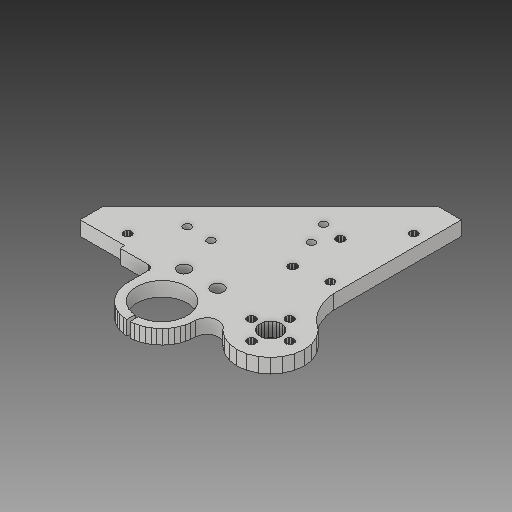
# Autodesk Inventor part: Left Bed Holder Lower
Saved by Autodesk Inventor 2018 (Build 220112000, 112)
## iProperties
Created: 2016-07-12
Part Number: Left Bed Holder Lower
Material: Generic
Document SubType Name: Modeling
Designer: joshmamo
Density: 1 g/cm^3
Appearance: Default
Author: joshmamo
Autodesk Inventor part; units mm, degrees
ref_plane "YZ Plane" through (0, 0, 0) normal (1, 0, 0) x (0, 1, 0)
ref_plane "XZ Plane" through (0, 0, 0) normal (0, 1, 0) x (-1, 0, 0)
ref_plane "XY Plane" through (0, 0, 0) normal (0, 0, 1) x (1, 0, 0)
sketch "Sketch2" plane through (0, 0, 0) normal (0, 1, 0) x (-1, 0, 0)
  line L0 (42.8996, 849.7412) -> (43.4826, 850.761)
  line L1 (43.4826, 850.761) -> (44.3097, 851.5953)
  line L2 (44.3097, 851.5953) -> (45.3245, 852.187)
  line L3 (45.3245, 852.187) -> (46.4579, 852.4959)
  line L4 (46.4579, 852.4959) -> (47.6326, 852.501)
  line L5 (47.6326, 852.501) -> (48.7686, 852.2018)
  line L6 (48.7686, 852.2018) -> (49.7885, 851.6188)
  line L7 (49.7885, 851.6188) -> (50.6227, 850.7917)
  line L8 (50.6227, 850.7917) -> (51.2145, 849.7769)
  line L9 (51.2145, 849.7769) -> (51.5234, 848.6435)
  line L10 (51.5234, 848.6435) -> (51.5284, 847.4688)
  line L11 (51.5284, 847.4688) -> (51.2293, 846.3328)
  line L12 (51.2293, 846.3328) -> (50.6463, 845.3129)
  line L13 (50.6463, 845.3129) -> (49.8192, 844.4787)
  line L14 (49.8192, 844.4787) -> (48.8044, 843.887)
  line L15 (48.8044, 843.887) -> (47.671, 843.578)
  line L16 (47.671, 843.578) -> (46.4963, 843.573)
  line L17 (46.4963, 843.573) -> (45.3603, 843.8722)
  line L18 (45.3603, 843.8722) -> (44.3404, 844.4551)
  line L19 (44.3404, 844.4551) -> (43.5062, 845.2822)
  line L20 (43.5062, 845.2822) -> (42.9144, 846.297)
  line L21 (42.9144, 846.297) -> (42.6055, 847.4304)
  line L22 (42.6055, 847.4304) -> (42.6005, 848.6052)
  line L23 (42.6005, 848.6052) -> (42.8996, 849.7412)
  line L24 (39.0644, 849.737) -> (39.5044, 849.6791)
  line L25 (39.5044, 849.6791) -> (39.9144, 849.5092)
  line L26 (39.9144, 849.5092) -> (40.2665, 849.2391)
  line L27 (40.2665, 849.2391) -> (40.5367, 848.887)
  line L28 (40.5367, 848.887) -> (40.7065, 848.477)
  line L29 (40.7065, 848.477) -> (40.7644, 848.037)
  line L30 (40.7644, 848.037) -> (40.7065, 847.597)
  line L31 (40.7065, 847.597) -> (40.5367, 847.187)
  line L32 (40.5367, 847.187) -> (40.2665, 846.8349)
  line L33 (40.2665, 846.8349) -> (39.9144, 846.5647)
  line L34 (39.9144, 846.5647) -> (39.5044, 846.3949)
  line L35 (39.5044, 846.3949) -> (39.0644, 846.337)
  line L36 (39.0644, 846.337) -> (38.6245, 846.3949)
  line L37 (38.6245, 846.3949) -> (38.2144, 846.5647)
  line L38 (38.2144, 846.5647) -> (37.8624, 846.8349)
  line L39 (37.8624, 846.8349) -> (37.5922, 847.187)
  line L40 (37.5922, 847.187) -> (37.4224, 847.597)
  line L41 (37.4224, 847.597) -> (37.3644, 848.037)
  line L42 (37.3644, 848.037) -> (37.4224, 848.477)
  line L43 (37.4224, 848.477) -> (37.5922, 848.887)
  line L44 (37.5922, 848.887) -> (37.8624, 849.2391)
  line L45 (37.8624, 849.2391) -> (38.2144, 849.5092)
  line L46 (38.2144, 849.5092) -> (38.6245, 849.6791)
  line L47 (38.6245, 849.6791) -> (39.0644, 849.737)
  line L48 (55.0644, 846.337) -> (54.6245, 846.3949)
  line L49 (54.6245, 846.3949) -> (54.2144, 846.5647)
  line L50 (54.2144, 846.5647) -> (53.8624, 846.8349)
  line L51 (53.8624, 846.8349) -> (53.5922, 847.187)
  line L52 (53.5922, 847.187) -> (53.4224, 847.597)
  line L53 (53.4224, 847.597) -> (53.3644, 848.037)
  line L54 (53.3644, 848.037) -> (53.4224, 848.477)
  line L55 (53.4224, 848.477) -> (53.5922, 848.887)
  line L56 (53.5922, 848.887) -> (53.8624, 849.2391)
  line L57 (53.8624, 849.2391) -> (54.2144, 849.5092)
  line L58 (54.2144, 849.5092) -> (54.6245, 849.6791)
  line L59 (54.6245, 849.6791) -> (55.0644, 849.737)
  line L60 (55.0644, 849.737) -> (55.5044, 849.6791)
  line L61 (55.5044, 849.6791) -> (55.9144, 849.5092)
  line L62 (55.9144, 849.5092) -> (56.2665, 849.2391)
  line L63 (56.2665, 849.2391) -> (56.5367, 848.887)
  line L64 (56.5367, 848.887) -> (56.7065, 848.477)
  line L65 (56.7065, 848.477) -> (56.7644, 848.037)
  line L66 (56.7644, 848.037) -> (56.7065, 847.597)
  line L67 (56.7065, 847.597) -> (56.5367, 847.187)
  line L68 (56.5367, 847.187) -> (56.2665, 846.8349)
  line L69 (56.2665, 846.8349) -> (55.9144, 846.5647)
  line L70 (55.9144, 846.5647) -> (55.5044, 846.3949)
  line L71 (55.5044, 846.3949) -> (55.0644, 846.337)
  line L72 (45.3644, 840.037) -> (45.4224, 840.477)
  line L73 (45.4224, 840.477) -> (45.5922, 840.887)
  line L74 (45.5922, 840.887) -> (45.8624, 841.2391)
  line L75 (45.8624, 841.2391) -> (46.2144, 841.5092)
  line L76 (46.2144, 841.5092) -> (46.6245, 841.6791)
  line L77 (46.6245, 841.6791) -> (47.0644, 841.737)
  line L78 (47.0644, 841.737) -> (47.5044, 841.6791)
  line L79 (47.5044, 841.6791) -> (47.9144, 841.5092)
  line L80 (47.9144, 841.5092) -> (48.2665, 841.2391)
  line L81 (48.2665, 841.2391) -> (48.5367, 840.887)
  line L82 (48.5367, 840.887) -> (48.7065, 840.477)
  line L83 (48.7065, 840.477) -> (48.7644, 840.037)
  line L84 (48.7644, 840.037) -> (48.7065, 839.597)
  line L85 (48.7065, 839.597) -> (48.5367, 839.187)
  line L86 (48.5367, 839.187) -> (48.2665, 838.8349)
  line L87 (48.2665, 838.8349) -> (47.9144, 838.5647)
  line L88 (47.9144, 838.5647) -> (47.5044, 838.3949)
  line L89 (47.5044, 838.3949) -> (47.0644, 838.337)
  line L90 (47.0644, 838.337) -> (46.6245, 838.3949)
  line L91 (46.6245, 838.3949) -> (46.2144, 838.5647)
  line L92 (46.2144, 838.5647) -> (45.8624, 838.8349)
  line L93 (45.8624, 838.8349) -> (45.5922, 839.187)
  line L94 (45.5922, 839.187) -> (45.4224, 839.597)
  line L95 (45.4224, 839.597) -> (45.3644, 840.037)
  line L96 (48.7644, 856.037) -> (48.7065, 855.597)
  line L97 (48.7065, 855.597) -> (48.5367, 855.187)
  line L98 (48.5367, 855.187) -> (48.2665, 854.8349)
  line L99 (48.2665, 854.8349) -> (47.9144, 854.5647)
  line L100 (47.9144, 854.5647) -> (47.5044, 854.3949)
  line L101 (47.5044, 854.3949) -> (47.0644, 854.337)
  line L102 (47.0644, 854.337) -> (46.6245, 854.3949)
  line L103 (46.6245, 854.3949) -> (46.2144, 854.5647)
  line L104 (46.2144, 854.5647) -> (45.8624, 854.8349)
  line L105 (45.8624, 854.8349) -> (45.5922, 855.187)
  line L106 (45.5922, 855.187) -> (45.4224, 855.597)
  line L107 (45.4224, 855.597) -> (45.3644, 856.037)
  line L108 (45.3644, 856.037) -> (45.4224, 856.477)
  line L109 (45.4224, 856.477) -> (45.5922, 856.887)
  line L110 (45.5922, 856.887) -> (45.8624, 857.2391)
  line L111 (45.8624, 857.2391) -> (46.2144, 857.5092)
  line L112 (46.2144, 857.5092) -> (46.6245, 857.6791)
  line L113 (46.6245, 857.6791) -> (47.0644, 857.737)
  line L114 (47.0644, 857.737) -> (47.5044, 857.6791)
  line L115 (47.5044, 857.6791) -> (47.9144, 857.5092)
  line L116 (47.9144, 857.5092) -> (48.2665, 857.2391)
  line L117 (48.2665, 857.2391) -> (48.5367, 856.887)
  line L118 (48.5367, 856.887) -> (48.7065, 856.477)
  line L119 (48.7065, 856.477) -> (48.7644, 856.037)
  line L120 (67.2644, 800.327) -> (67.2065, 799.887)
  line L121 (67.2065, 799.887) -> (67.0367, 799.477)
  line L122 (67.0367, 799.477) -> (66.7665, 799.1249)
  line L123 (66.7665, 799.1249) -> (66.4144, 798.8547)
  line L124 (66.4144, 798.8547) -> (66.0044, 798.6849)
  line L125 (66.0044, 798.6849) -> (65.5644, 798.627)
  line L126 (65.5644, 798.627) -> (65.1245, 798.6849)
  line L127 (65.1245, 798.6849) -> (64.7144, 798.8547)
  line L128 (64.7144, 798.8547) -> (64.3624, 799.1249)
  line L129 (64.3624, 799.1249) -> (64.0922, 799.477)
  line L130 (64.0922, 799.477) -> (63.9224, 799.887)
  line L131 (63.9224, 799.887) -> (63.8644, 800.327)
  line L132 (63.8644, 800.327) -> (63.9224, 800.7669)
  line L133 (63.9224, 800.7669) -> (64.0922, 801.177)
  line L134 (64.0922, 801.177) -> (64.3624, 801.529)
  line L135 (64.3624, 801.529) -> (64.7144, 801.7992)
  line L136 (64.7144, 801.7992) -> (65.1245, 801.969)
  line L137 (65.1245, 801.969) -> (65.5644, 802.027)
  line L138 (65.5644, 802.027) -> (66.0044, 801.969)
  line L139 (66.0044, 801.969) -> (66.4144, 801.7992)
  line L140 (66.4144, 801.7992) -> (66.7665, 801.529)
  line L141 (66.7665, 801.529) -> (67.0367, 801.177)
  line L142 (67.0367, 801.177) -> (67.2065, 800.7669)
  line L143 (67.2065, 800.7669) -> (67.2644, 800.327)
  line L144 (66.4144, 818.8547) -> (66.0044, 818.6849)
  line L145 (66.0044, 818.6849) -> (65.5644, 818.627)
  line L146 (65.5644, 818.627) -> (65.1245, 818.6849)
  line L147 (65.1245, 818.6849) -> (64.7144, 818.8547)
  line L148 (64.7144, 818.8547) -> (64.3624, 819.1249)
  line L149 (64.3624, 819.1249) -> (64.0922, 819.477)
  line L150 (64.0922, 819.477) -> (63.9224, 819.887)
  line L151 (63.9224, 819.887) -> (63.8644, 820.327)
  line L152 (63.8644, 820.327) -> (63.9224, 820.7669)
  line L153 (63.9224, 820.7669) -> (64.0922, 821.177)
  line L154 (64.0922, 821.177) -> (64.3624, 821.529)
  line L155 (64.3624, 821.529) -> (64.7144, 821.7992)
  line L156 (64.7144, 821.7992) -> (65.1245, 821.969)
  line L157 (65.1245, 821.969) -> (65.5644, 822.027)
  line L158 (65.5644, 822.027) -> (66.0044, 821.969)
  line L159 (66.0044, 821.969) -> (66.4144, 821.7992)
  line L160 (66.4144, 821.7992) -> (66.7665, 821.529)
  line L161 (66.7665, 821.529) -> (67.0367, 821.177)
  line L162 (67.0367, 821.177) -> (67.2065, 820.7669)
  line L163 (67.2065, 820.7669) -> (67.2644, 820.327)
  line L164 (67.2644, 820.327) -> (67.2065, 819.887)
  line L165 (67.2065, 819.887) -> (67.0367, 819.477)
  line L166 (67.0367, 819.477) -> (66.7665, 819.1249)
  line L167 (66.7665, 819.1249) -> (66.4144, 818.8547)
  line L168 (52.4786, 816.4915) -> (52.0644, 816.437)
  line L169 (52.0644, 816.437) -> (51.6503, 816.4915)
  line L170 (51.6503, 816.4915) -> (51.2644, 816.6513)
  line L171 (51.2644, 816.6513) -> (50.9331, 816.9056)
  line L172 (50.9331, 816.9056) -> (50.6788, 817.237)
  line L173 (50.6788, 817.237) -> (50.519, 817.6229)
  line L174 (50.519, 817.6229) -> (50.4644, 818.037)
  line L175 (50.4644, 818.037) -> (50.519, 818.4511)
  line L176 (50.519, 818.4511) -> (50.6788, 818.837)
  line L177 (50.6788, 818.837) -> (50.9331, 819.1683)
  line L178 (50.9331, 819.1683) -> (51.2644, 819.4226)
  line L179 (51.2644, 819.4226) -> (51.6503, 819.5825)
  line L180 (51.6503, 819.5825) -> (52.0644, 819.637)
  line L181 (52.0644, 819.637) -> (52.4786, 819.5825)
  line L182 (52.4786, 819.5825) -> (52.8644, 819.4226)
  line L183 (52.8644, 819.4226) -> (53.1958, 819.1683)
  line L184 (53.1958, 819.1683) -> (53.4501, 818.837)
  line L185 (53.4501, 818.837) -> (53.6099, 818.4511)
  line L186 (53.6099, 818.4511) -> (53.6644, 818.037)
  line L187 (53.6644, 818.037) -> (53.6099, 817.6229)
  line L188 (53.6099, 817.6229) -> (53.4501, 817.237)
  line L189 (53.4501, 817.237) -> (53.1958, 816.9056)
  line L190 (53.1958, 816.9056) -> (52.8644, 816.6513)
  line L191 (52.8644, 816.6513) -> (52.4786, 816.4915)
  line L192 (113.6099, 843.4511) -> (113.6644, 843.037)
  line L193 (113.6644, 843.037) -> (113.6099, 842.6229)
  line L194 (113.6099, 842.6229) -> (113.4501, 842.237)
  line L195 (113.4501, 842.237) -> (113.1958, 841.9056)
  line L196 (113.1958, 841.9056) -> (112.8644, 841.6513)
  line L197 (112.8644, 841.6513) -> (112.4786, 841.4915)
  line L198 (112.4786, 841.4915) -> (112.0644, 841.437)
  line L199 (112.0644, 841.437) -> (111.6503, 841.4915)
  line L200 (111.6503, 841.4915) -> (111.2644, 841.6513)
  line L201 (111.2644, 841.6513) -> (110.9331, 841.9056)
  line L202 (110.9331, 841.9056) -> (110.6788, 842.237)
  line L203 (110.6788, 842.237) -> (110.519, 842.6229)
  line L204 (110.519, 842.6229) -> (110.4644, 843.037)
  line L205 (110.4644, 843.037) -> (110.519, 843.4511)
  line L206 (110.519, 843.4511) -> (110.6788, 843.837)
  line L207 (110.6788, 843.837) -> (110.9331, 844.1683)
  line L208 (110.9331, 844.1683) -> (111.2644, 844.4226)
  line L209 (111.2644, 844.4226) -> (111.6503, 844.5825)
  line L210 (111.6503, 844.5825) -> (112.0644, 844.637)
  line L211 (112.0644, 844.637) -> (112.4786, 844.5825)
  line L212 (112.4786, 844.5825) -> (112.8644, 844.4226)
  line L213 (112.8644, 844.4226) -> (113.1958, 844.1683)
  line L214 (113.1958, 844.1683) -> (113.4501, 843.837)
  line L215 (113.4501, 843.837) -> (113.6099, 843.4511)
  line L216 (52.4786, 781.4915) -> (52.0644, 781.437)
  line L217 (52.0644, 781.437) -> (51.6503, 781.4915)
  line L218 (51.6503, 781.4915) -> (51.2644, 781.6513)
  line L219 (51.2644, 781.6513) -> (50.9331, 781.9056)
  line L220 (50.9331, 781.9056) -> (50.6788, 782.237)
  line L221 (50.6788, 782.237) -> (50.519, 782.6229)
  line L222 (50.519, 782.6229) -> (50.4644, 783.037)
  line L223 (50.4644, 783.037) -> (50.519, 783.4511)
  line L224 (50.519, 783.4511) -> (50.6788, 783.837)
  line L225 (50.6788, 783.837) -> (50.9331, 784.1683)
  line L226 (50.9331, 784.1683) -> (51.2644, 784.4226)
  line L227 (51.2644, 784.4226) -> (51.6503, 784.5825)
  line L228 (51.6503, 784.5825) -> (52.0644, 784.637)
  line L229 (52.0644, 784.637) -> (52.4786, 784.5825)
  line L230 (52.4786, 784.5825) -> (52.8644, 784.4226)
  line L231 (52.8644, 784.4226) -> (53.1958, 784.1683)
  line L232 (53.1958, 784.1683) -> (53.4501, 783.837)
  line L233 (53.4501, 783.837) -> (53.6099, 783.4511)
  line L234 (53.6099, 783.4511) -> (53.6644, 783.037)
  line L235 (53.6644, 783.037) -> (53.6099, 782.6229)
  line L236 (53.6099, 782.6229) -> (53.4501, 782.237)
  line L237 (53.4501, 782.237) -> (53.1958, 781.9056)
  line L238 (53.1958, 781.9056) -> (52.8644, 781.6513)
  line L239 (52.8644, 781.6513) -> (52.4786, 781.4915)
  line L240 (127.0877, 838.0325) -> (127.0877, 847.9749)
  line L241 (127.0877, 847.9749) -> (108.3077, 847.9749)
  line L242 (108.3077, 847.9749) -> (108.3077, 849.9151)
  line L243 (108.3077, 849.9151) -> (96.4077, 849.9151)
  line L244 (96.4077, 849.9151) -> (96.043, 849.947)
  line L245 (96.043, 849.947) -> (95.3846, 850.254)
  line L246 (95.3846, 850.254) -> (95.0847, 850.464)
  line L247 (95.0847, 850.464) -> (94.8259, 850.7228)
  line L248 (94.8259, 850.7228) -> (94.6159, 851.0227)
  line L249 (94.6159, 851.0227) -> (94.4612, 851.3544)
  line L250 (94.4612, 851.3544) -> (94.3665, 851.708)
  line L251 (94.3665, 851.708) -> (94.3346, 852.0727)
  line L252 (94.3346, 852.0727) -> (94.3346, 860.4727)
  line L253 (94.3346, 860.4727) -> (94.2223, 862.2422)
  line L254 (94.2223, 862.2422) -> (93.8873, 863.9833)
  line L255 (93.8873, 863.9833) -> (93.3349, 865.6681)
  line L256 (93.3349, 865.6681) -> (92.5739, 867.2696)
  line L257 (92.5739, 867.2696) -> (91.6167, 868.762)
  line L258 (91.6167, 868.762) -> (90.4785, 870.1215)
  line L259 (90.4785, 870.1215) -> (89.1776, 871.3262)
  line L260 (89.1776, 871.3262) -> (87.7349, 872.3569)
  line L261 (87.7349, 872.3569) -> (86.1735, 873.197)
  line L262 (86.1735, 873.197) -> (84.5184, 873.8329)
  line L263 (84.5184, 873.8329) -> (82.7962, 874.2546)
  line L264 (82.7962, 874.2546) -> (81.0346, 874.4552)
  line L265 (81.0346, 874.4552) -> (81.0346, 870.9493)
  line L266 (81.0346, 870.9493) -> (82.6711, 870.7094)
  line L267 (82.6711, 870.7094) -> (84.2496, 870.2155)
  line L268 (84.2496, 870.2155) -> (85.731, 869.4798)
  line L269 (85.731, 869.4798) -> (87.0784, 868.5207)
  line L270 (87.0784, 868.5207) -> (88.2586, 867.3618)
  line L271 (88.2586, 867.3618) -> (89.2421, 866.032)
  line L272 (89.2421, 866.032) -> (90.0046, 864.5643)
  line L273 (90.0046, 864.5643) -> (90.5271, 862.995)
  line L274 (90.5271, 862.995) -> (90.7967, 861.3631)
  line L275 (90.7967, 861.3631) -> (90.8068, 859.7092)
  line L276 (90.8068, 859.7092) -> (90.5569, 858.0742)
  line L277 (90.5569, 858.0742) -> (90.0535, 856.4987)
  line L278 (90.0535, 856.4987) -> (89.3088, 855.0218)
  line L279 (89.3088, 855.0218) -> (88.3415, 853.6801)
  line L280 (88.3415, 853.6801) -> (87.1755, 852.5071)
  line L281 (87.1755, 852.5071) -> (85.8398, 851.5316)
  line L282 (85.8398, 851.5316) -> (84.3674, 850.778)
  line L283 (84.3674, 850.778) -> (82.795, 850.265)
  line L284 (82.795, 850.265) -> (81.1615, 850.0053)
  line L285 (81.1615, 850.0053) -> (79.5076, 850.0053)
  line L286 (79.5076, 850.0053) -> (77.8741, 850.265)
  line L287 (77.8741, 850.265) -> (76.3017, 850.778)
  line L288 (76.3017, 850.778) -> (74.8293, 851.5316)
  line L289 (74.8293, 851.5316) -> (73.4936, 852.5071)
  line L290 (73.4936, 852.5071) -> (72.3276, 853.6801)
  line L291 (72.3276, 853.6801) -> (71.3603, 855.0218)
  line L292 (71.3603, 855.0218) -> (70.6156, 856.4987)
  line L293 (70.6156, 856.4987) -> (70.1122, 858.0742)
  line L294 (70.1122, 858.0742) -> (69.8623, 859.7092)
  line L295 (69.8623, 859.7092) -> (69.8724, 861.3631)
  line L296 (69.8724, 861.3631) -> (70.142, 862.995)
  line L297 (70.142, 862.995) -> (70.6646, 864.5643)
  line L298 (70.6646, 864.5643) -> (71.427, 866.032)
  line L299 (71.427, 866.032) -> (72.4106, 867.3618)
  line L300 (72.4106, 867.3618) -> (73.5907, 868.5207)
  line L301 (73.5907, 868.5207) -> (74.9382, 869.4798)
  line L302 (74.9382, 869.4798) -> (76.4195, 870.2155)
  line L303 (76.4195, 870.2155) -> (77.9981, 870.7094)
  line L304 (77.9981, 870.7094) -> (79.6346, 870.9493)
  line L305 (79.6346, 870.9493) -> (79.6346, 874.4552)
  line L306 (79.6346, 874.4552) -> (77.8729, 874.2546)
  line L307 (77.8729, 874.2546) -> (76.1507, 873.8329)
  line L308 (76.1507, 873.8329) -> (74.4956, 873.197)
  line L309 (74.4956, 873.197) -> (72.9342, 872.3569)
  line L310 (72.9342, 872.3569) -> (71.4915, 871.3262)
  line L311 (71.4915, 871.3262) -> (70.1906, 870.1215)
  line L312 (70.1906, 870.1215) -> (69.0524, 868.762)
  line L313 (69.0524, 868.762) -> (68.0952, 867.2696)
  line L314 (68.0952, 867.2696) -> (67.3343, 865.6681)
  line L315 (67.3343, 865.6681) -> (66.7819, 863.9833)
  line L316 (66.7819, 863.9833) -> (66.4468, 862.2422)
  line L317 (66.4468, 862.2422) -> (66.3346, 860.4727)
  arc A0 (57.9592, 856.9316) -> (66.3346, 860.4727) centre (61.3983, 860.4727) ccw
  line L318 (57.9592, 856.9316) -> (57.0877, 858.0673)
  line L319 (57.0877, 858.0673) -> (54.1588, 860.3147)
  line L320 (54.1588, 860.3147) -> (50.748, 861.7275)
  line L321 (50.748, 861.7275) -> (47.0877, 862.2094)
  line L322 (47.0877, 862.2094) -> (43.4275, 861.7275)
  line L323 (43.4275, 861.7275) -> (40.0166, 860.3147)
  line L324 (40.0166, 860.3147) -> (37.0877, 858.0673)
  line L325 (37.0877, 858.0673) -> (34.8403, 855.1384)
  line L326 (34.8403, 855.1384) -> (33.4275, 851.7275)
  line L327 (33.4275, 851.7275) -> (32.9456, 848.0673)
  line L328 (32.9456, 848.0673) -> (33.4275, 844.407)
  line L329 (33.4275, 844.407) -> (34.8403, 840.9962)
  line L330 (34.8403, 840.9962) -> (37.0877, 838.0673)
  line L331 (37.0877, 838.0673) -> (39.0184, 836.5858)
  arc A1 (47.0644, 821.7992) -> (39.0184, 836.5858) centre (26.3948, 820.1343) ccw
  line L332 (47.0644, 821.7992) -> (47.0644, 768.0325)
  line L333 (47.0644, 768.0325) -> (57.0877, 768.0325)
  line L334 (57.0877, 768.0325) -> (127.0877, 838.0325)
  circle A2 centre (102.0877, 828.0325) radius 1.6
  circle A3 centre (92.0877, 828.0325) radius 1.6
  circle A4 centre (74.4298, 798.5685) radius 1.6
  circle A5 centre (70.3783, 807.7111) radius 1.6
  circle A6 centre (87.3346, 844.0325) radius 2.6
  circle A7 centre (73.3346, 844.0325) radius 2.6
  point P0 (0, 0)
  constraints: 670 end point, 8 centre point, 4 point on circle
extrude "Extrusion1" add sketch "Sketch2" along normal blind 6
sketch "Sketch4" plane through (0, 6, 0) normal (0, 1, 0) x (1, 0, 0)
  arc A0 (-79.6346, -870.9288) -> (-81.0346, -870.9288) centre (-80.3346, -860.3519) ccw
  point P0 (0, 0)
  constraints: 2 point on circle, 1 centre point
hole "Hole1" at (-80.3346, 6, 860.3519) direction (0, -1, 0) diameter 21.2 depth 8 tip angle 118
body "Solid1"
